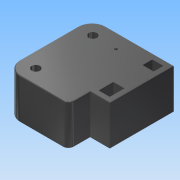
# Autodesk Inventor part: датчик  окончания филамента
Saved by Autodesk Inventor 2017 (Build 210142000, 142)
## iProperties
Part Number: датчик  окончания филамента
Material: Типовые
Document SubType Name: Modeling
Designer: Max
Mass: 11.791 g
Surface Area: 44.4124 cm^2
Volume: 11.791 cm^3
Density: 1 g/cm^3
Appearance: Цинк
Author: Max
Autodesk Inventor part; units mm, degrees
ref_plane "YZ Plane" through (0, 0, 0) normal (1, 0, 0) x (0, 1, 0)
ref_plane "XZ Plane" through (0, 0, 0) normal (0, 1, 0) x (-1, 0, 0)
ref_plane "XY Plane" through (0, 0, 0) normal (0, 0, 1) x (1, 0, 0)
sketch "Эскиз1" plane through (0, 0, 0) normal (0, 0, 1) x (1, 0, 0)
  line L0 (5, 0) -> (22.5, 0)
  line L1 (29.6, 7.88) -> (29.6, 31)
  line L2 (29.6, 31) -> (5, 31)
  line L3 (0, 26) -> (0, 5)
  line L4 (29.6, 7.88) -> (22.5, 7.88)
  line L5 (22.5, 7.88) -> (22.5, 0)
  line L6 (23.81, 9.63) -> (27.81, 9.63)
  line L7 (27.81, 9.63) -> (27.81, 14.93)
  line L8 (27.81, 14.93) -> (23.81, 14.93)
  line L9 (23.81, 14.93) -> (23.81, 9.63)
  line L10 (23.81, 25.53) -> (27.81, 25.53)
  line L11 (27.81, 25.53) -> (27.81, 29.03)
  line L12 (27.81, 29.03) -> (23.81, 29.03)
  line L13 (23.81, 29.03) -> (23.81, 25.53)
  arc A0 (0, 5) -> (5, 0) centre (5, 5) ccw
  arc A1 (5, 31) -> (0, 26) centre (5, 26) ccw
  circle A2 centre (5.5, 5.2) radius 1.5
  circle A3 centre (5.5, 25.8) radius 1.5
  circle A4 centre (14, 25.7) radius 0.5
  line L14 (14, 25.7) -> (14, 9.2355) construction
  line L15 (14, 21) -> (16.5, 17)
  line L16 (16.5, 17) -> (15.25, 17)
  line L17 (15.25, 17) -> (15.25, 11.2)
  line L18 (15.25, 11.2) -> (12.75, 11.2)
  line L19 (12.75, 11.2) -> (12.75, 17)
  line L20 (12.75, 17) -> (11.5, 17)
  line L21 (11.5, 17) -> (14, 21)
  point P0 (0, 0)
  dimension "d0" = 31
  dimension "d1" = 29.6
  dimension "d2" = 23.12
  dimension "d3" = 22.5
  dimension "d4" = 4
  dimension "d5" = 5.3
  dimension "d6" = 3.5
  dimension "d7" = 4
  dimension "d8" = 1.75
  dimension "d9" = 1.79
  dimension "d10" = 10.6
  dimension "d11" = 5
  dimension "d12" = 3
  dimension "d13" = 3
  dimension "d14" = 5.5
  dimension "d15" = 5.5
  dimension "d16" = 5.2
  dimension "d17" = 5.2
  dimension "d18" = 3.7
  dimension "d23" = 1
  dimension "d24" = 5.3
  dimension "d25" = 15.6
  dimension "d26" = 9.8
  dimension "d27" = 2.5
  dimension "d28" = 5
  dimension "d29" = 4
  dimension "d30" = 10
  constraints: 44 end point, 7 point on line, 6 parallel, 6 perpendicular, 5 centre point, 4 horizontal, 4 point on circle, 4 tangent, 1 equal radius, 1 vertical, 2 other
  measures "d0" distance between parallel lines of L0 L2
  measures "d1" distance between parallel lines of L1 L3
  measures "d2" distance between parallel lines of L2 L4
  measures "d3" distance between parallel lines of L3 L5
  measures "d4" distance between parallel lines of L7 L9
  measures "d5" distance between parallel lines of L6 L8
  measures "d6" distance between parallel lines of L12 L10
  measures "d7" distance between parallel lines of L11 L13
  measures "d8" distance between parallel lines of L4 L6
  measures "d9" distance between parallel lines of L1 L7
  measures "d10" distance between parallel lines of L8 L10
  measures "d11" radius of A0
  measures "d12" diameter of A2
  measures "d13" diameter of A3
  measures "d14" distance from line of L3 A3.centre
  measures "d15" distance from line of L3 A2.centre
  measures "d16" distance from line of L0 A2.centre
  measures "d17" distance from line of A3.centre L2
  measures "d18" distance edge to line of A3 L2
  measures "d23" diameter of A4
  measures "d24" distance from line of L2 L14.start
  measures "d25" distance from line of L1 L14.start
  measures "d26" distance from line of L15.start L18
  measures "d27" distance between parallel lines of L17 L19
  measures "d28" distance of L15.end L20.end
  measures "d29" distance from line of L16 L15.start
  measures "d30" distance from line of L2 L15.start
extrude "Выдавливание1" add sketch "Эскиз1" along normal mid plane 14.6
fillet "Сопряжение1" radius 2 1 edges at (22.5, 0, 0)
fillet "Сопряжение2" radius 0.3 18 edges at (1.4645, 29.5355, 7.3) (0, 15.5, 7.3) (1.4645, 1.4645, 7.3) (12.75, 0, 7.3) (21.9142, 0.5858, 7.3) (22.5, 4.94, 7.3) (17.3, 31, 7.3) (29.6, 19.44, 7.3) (26.05, 7.88, 7.3) (29.6, 19.44, -7.3) (26.05, 7.88, -7.3) (21.9142, 0.5858, -7.3) (12.75, 0, -7.3) (1.4645, 1.4645, -7.3) (0, 15.5, -7.3) (1.4645, 29.5355, -7.3) (17.3, 31, -7.3) (22.5, 4.94, -7.3)
extrude "Выдавливание2" add sketch "Эскиз1" along normal mid plane 14 contours L15 L16 L17 L18 L19 L20 L21
fillet "Сопряжение3" radius 0.3 7 edges at (12.75, 19, 7.3) (12.125, 17, 7.3) (12.75, 14.1, 7.3) (14, 11.2, 7.3) (15.25, 14.1, 7.3) (15.875, 17, 7.3) (15.25, 19, 7.3)
sketch "Эскиз2" plane through (5, 31, -7) normal (0, 1, 0) x (1, 0, 0)
  line L0 (-5, -7) -> (24.6, -7) construction
  line L1 (24.6, 0) -> (24.6, -14) construction
  circle A0 centre (20.6, -7) radius 1
  circle A1 centre (20.6, -7) radius 4
  dimension "d34" = 2
  dimension "d35" = 8
  constraints: 2 centre point, 2 end point, 1 coincident, 1 midpoint, 1 point on line, 1 tangent
  measures "d34" diameter of A0
  measures "d35" diameter of A1
extrude "Выдавливание3" add sketch "Эскиз2" against normal blind 23.12 and the other way blind 3.4
fillet "Сопряжение4" radius 0.3 1 edges at (21.6, 34.4, 0)
extrude "Выдавливание4" cut sketch "Эскиз2" along normal mid plane 50 contours A0
fillet "Сопряжение5" radius 0.3 3 edges at (29.5121, 7.9679, -7.2121) (29.5121, 7.9679, 7.2121) (29.6, 7.88, 0)
fillet "Сопряжение6" radius 0.3 4 edges at (29.5121, 30.9121, 7.2121) (29.6, 31, 3.5) (29.5121, 30.9121, -7.2121) (29.6, 31, -3.5)
sketch "Эскиз3" plane through (5, 0, -7) normal (0, -1, 0) x (1, 0, 0)
  line L0 (12.4, 12.5) -> (6.4, 12.5)
  line L1 (6.4, 12.5) -> (6.4, 1.5)
  line L2 (6.4, 1.5) -> (12.4, 1.5)
  line L3 (12.4, 1.5) -> (12.4, 12.5)
  line L4 (-5, 14) -> (-5, 0) projected
  line L5 (0, 14) -> (15.5, 14) projected
  line L6 (7.75, 0) -> (10.25, 0) projected
  line L7 (15.5, 14.3) -> (0, 14.3) projected
  line L8 (12.2, 12.3) -> (6.6, 12.3)
  line L9 (6.6, 12.3) -> (6.6, 1.7)
  line L10 (6.6, 1.7) -> (12.2, 1.7)
  line L11 (12.2, 1.7) -> (12.2, 12.3)
  line L12 (12.2, 9.5) -> (11.5, 9.5)
  line L13 (11.5, 9.5) -> (11.5, 8.7)
  line L14 (11.5, 8.7) -> (12.2, 8.7)
  line L15 (12.2, 8.7) -> (12.2, 9.5)
  line L16 (12.2, 5.3) -> (11.5, 5.3)
  line L17 (11.5, 5.3) -> (11.5, 4.5)
  line L18 (11.5, 4.5) -> (12.2, 4.5)
  line L19 (12.2, 4.5) -> (12.2, 5.3)
  line L20 (12.2, 7) -> (7.2247, 7) construction
  line L21 (11.5, 12.3) -> (11.5, 1.7)
  line L22 (11.5, 12.3) -> (12.2, 12.3)
  line L23 (12.2, 12.3) -> (12.2, 1.7)
  line L24 (12.2, 1.7) -> (11.5, 1.7)
  line L25 (11.5, 1.7) -> (11.5, 12.3)
  line L26 (11, 12.3) -> (6.6, 12.3)
  line L27 (6.6, 12.3) -> (6.6, 11.6)
  line L28 (6.6, 11.6) -> (11, 11.6)
  line L29 (11, 11.6) -> (11, 12.3)
  line L30 (11, 1.7) -> (6.6, 1.7)
  line L31 (6.6, 1.7) -> (6.6, 2.4)
  line L32 (6.6, 2.4) -> (11, 2.4)
  line L33 (11, 2.4) -> (11, 1.7)
  line L34 (7.3, 11.6) -> (6.6, 11.6)
  line L35 (6.6, 11.6) -> (6.6, 2.4)
  line L36 (6.6, 2.4) -> (7.3, 2.4)
  line L37 (7.3, 2.4) -> (7.3, 11.6)
  line L38 (10.25, 10.3107) -> (9.7123, 10.3107)
  line L39 (9.7123, 10.3107) -> (9.7123, 9.5)
  line L40 (9.7123, 9.5) -> (10.25, 9.5)
  line L41 (10.25, 9.5) -> (10.25, 10.3107)
  line L42 (10.25, 7.4336) -> (9.7123, 7.4336)
  line L43 (9.7123, 7.4336) -> (9.7123, 6.5705)
  line L44 (9.7123, 6.5705) -> (10.25, 6.5705)
  line L45 (10.25, 6.5705) -> (10.25, 7.4336)
  line L46 (10.25, 4.6411) -> (9.7123, 4.6411)
  line L47 (9.7123, 4.6411) -> (9.7123, 3.8288)
  line L48 (9.7123, 3.8288) -> (10.25, 3.8288)
  line L49 (10.25, 3.8288) -> (10.25, 4.6411)
  point P0 (-5, 7)
  dimension "d45" = 11.4
  dimension "d46" = 1.5
  dimension "d47" = 1.5
  dimension "d48" = 1.8
  dimension "d49" = 6
  dimension "d50" = 0.2
  dimension "d51" = 0.7
  dimension "d52" = 5
  dimension "d53" = 0.8
  dimension "d54" = 0.7
  dimension "d55" = 0.7
  dimension "d56" = 0.7
  dimension "d57" = 0.5
  dimension "d58" = 0.5
  constraints: 92 end point, 22 parallel, 14 point on line, 12 perpendicular, 11 horizontal, 1 collinear, 1 midpoint, 5 other
  measures "d45" distance between parallel lines of L4 L1
  measures "d46" distance between parallel lines of L5 L0
  measures "d47" distance between parallel lines of L6 L2
  measures "d48" distance between parallel lines of L0 L7
  measures "d49" distance between parallel lines of L3 L1
  measures "d50" distance between parallel lines of L3 L11
  measures "d51" distance between parallel lines of L11 L21
  measures "d52" distance between parallel lines of L18 L12
  measures "d53" distance between parallel lines of L12 L14
  measures "d54" distance between parallel lines of L26 L28
  measures "d55" distance between parallel lines of L10 L32
  measures "d56" distance between parallel lines of L35 L37
  measures "d57" distance between parallel lines of L21 L29
  measures "d58" distance between parallel lines of L33 L21
extrude "Выдавливание5" cut sketch "Эскиз3" against normal blind 1 contours L3 L2 L1 L0
extrude "Выдавливание6" cut sketch "Эскиз3" against normal blind 5.6 contours L21 L13 L17 L10 L33 L32 L37 L28 L29 L8
extrude "Выдавливание7" cut sketch "Эскиз3" against normal blind 4 contours L11 L14 L13 L12 | L11 L18 L17 L16
